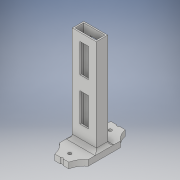
# Autodesk Inventor part: Pizza1
Saved by Autodesk Inventor 2018.2 (Build 222227000, 227)
## iProperties
Created: 2018-03-29
Part Number: Pizza1
Material: Generic
Document SubType Name: Modeling
Designer: MIABo
Density: 1 g/cm^3
Appearance: Default
Author: MIABo
## iProperties of the stored document Pizza1_3DPrint.ipt
Created: 2018-03-29
Part Number: Pizza1_3DPrint
Material: Generic
Document SubType Name: Modeling
Designer: MIABo
Density: 1 g/cm^3
Appearance: Default
Author: MIABo
Autodesk Inventor part; units mm, degrees
ref_plane "YZ Plane" through (0, 0, 0) normal (1, 0, 0) x (0, 1, 0)
ref_plane "XZ Plane" through (0, 0, 0) normal (0, 1, 0) x (-1, 0, 0)
ref_plane "XY Plane" through (0, 0, 0) normal (0, 0, 1) x (1, 0, 0)
sketch "Sketch1" plane through (0, 0, 0) normal (0, 1, 0) x (-1, 0, 0)
  line L0 (12.7, 33.3375) -> (-12.7, 33.3375)
  line L1 (-12.7, 33.3375) -> (-12.7, -33.3375)
  line L2 (-12.7, -33.3375) -> (12.7, -33.3375)
  line L3 (12.7, -33.3375) -> (12.7, 33.3375)
  line L4 (12.7, 33.3375) -> (-12.7, -33.3375) construction
  line L5 (-12.7, 33.3375) -> (12.7, -33.3375) construction
  point P0 (0, 0)
  dimension "d0" = 25.4
  dimension "d1" = 66.675
  constraints: 12 end point, 2 midpoint, 2 parallel, 1 horizontal, 1 perpendicular
  measures "d0" distance of L2.end L1.end
  measures "d1" distance of L1.end L0.end
extrude "Extrusion1" add sketch "Sketch1" along normal blind 5.08
sketch "Sketch3" plane through (0, 5.08, 0) normal (0, 1, 0) x (1, 0, 0)
  line L0 (-10.541, 5.08) -> (10.541, 5.08)
  line L1 (10.541, 5.08) -> (10.541, -5.08)
  line L2 (10.541, -5.08) -> (-10.541, -5.08)
  line L3 (-10.541, -5.08) -> (-10.541, 5.08)
  line L4 (-10.541, 5.08) -> (10.541, -5.08) construction
  line L5 (10.541, 5.08) -> (-10.541, -5.08) construction
  point P0 (0, 0)
  dimension "d8" = 21.082
  dimension "d9" = 10.16
  constraints: 12 end point, 2 midpoint, 2 parallel, 1 horizontal, 1 perpendicular
  measures "d8" distance of L1.end L2.end
  measures "d9" distance of L0.end L1.end
extrude "Extrusion3" add sketch "Sketch3" along normal blind 96.8375
sketch "Sketch2" plane through (0, 5.08, 0) normal (0, 1, 0) x (1, 0, 0)
  line L0 (-9.271, -3.81) -> (9.271, -3.81)
  line L1 (9.271, -3.81) -> (9.271, 3.81)
  line L2 (9.271, 3.81) -> (-9.271, 3.81)
  line L3 (-9.271, 3.81) -> (-9.271, -3.81)
  line L4 (-9.271, -3.81) -> (9.271, 3.81) construction
  line L5 (9.271, -3.81) -> (-9.271, 3.81) construction
  point P0 (0, 0)
  dimension "d4" = 18.542
  dimension "d5" = 7.62
  constraints: 12 end point, 2 midpoint, 2 parallel, 1 horizontal, 1 perpendicular
  measures "d4" distance of L2.end L1.end
  measures "d5" distance of L1.end L0.end
extrude "Extrusion2" cut sketch "Sketch2" along normal through all both and the other way through all
fillet "Fillet1" radius 3.175 4 edges at (0, 5.08, 5.08) (10.541, 5.08, 0) (0, 5.08, -5.08) (-10.541, 5.08, 0)
sketch "Sketch5" plane through (0, 101.9175, 0) normal (0, 1, 0) x (1, 0, 0)
  line L0 (-19.05, 12.7) -> (19.05, 12.7)
  line L1 (19.05, 12.7) -> (19.05, -12.7)
  line L2 (19.05, -12.7) -> (-19.05, -12.7)
  line L3 (-19.05, -12.7) -> (-19.05, 12.7)
  line L4 (-19.05, 12.7) -> (19.05, -12.7) construction
  line L5 (19.05, 12.7) -> (-19.05, -12.7) construction
  point P0 (0, 0)
  constraints: 12 end point, 2 midpoint, 2 parallel, 1 horizontal, 1 perpendicular
extrude "Extrusion5" cut sketch "Sketch5" against normal blind 12.7
sketch "Sketch6" plane through (0, 5.08, 0) normal (0, 1, 0) x (1, 0, 0)
  point P0 (0, 0)
sketch "Sketch7" plane through (0, 5.08, 0) normal (0, 1, 0) x (1, 0, 0)
  line L0 (12.7, 33.3375) -> (-12.7, 33.3375) projected
  line L1 (12.7, -33.3375) -> (12.7, 33.3375) projected
  arc A0 (6.35, 33.3375) -> (12.7, 14.0352) centre (24.8324, 28.7221) ccw
  line L2 (-12.7, 33.3375) -> (-12.7, -33.3375) projected
  arc A1 (-12.7, 14.0352) -> (-6.35, 33.3375) centre (-24.8324, 28.7221) ccw
  line L3 (-12.7, -33.3375) -> (12.7, -33.3375) projected
  arc A2 (-6.35, -33.3375) -> (-12.7, -14.0352) centre (-24.8324, -28.7221) ccw
  arc A3 (12.7, -14.0352) -> (6.35, -33.3375) centre (24.8324, -28.7221) ccw
  line L4 (12.7, -14.0352) -> (12.7, -33.3375)
  line L5 (12.7, -33.3375) -> (6.35, -33.3375)
  line L6 (-6.35, -33.3375) -> (-12.7, -33.3375)
  line L7 (-12.7, -14.0352) -> (-12.7, -33.3375)
  line L8 (-12.7, 14.0352) -> (-12.7, 33.3375)
  line L9 (-6.35, 33.3375) -> (-12.7, 33.3375)
  line L10 (6.35, 33.3375) -> (12.7, 33.3375)
  line L11 (12.7, 14.0352) -> (12.7, 33.3375)
  point P0 (0, 0)
  dimension "d62" = 20.32
  dimension "d63" = 19.05
  dimension "d64" = 20.32
  dimension "d65" = 19.05
  dimension "d68" = 20.32
  dimension "d69" = 19.05
  dimension "d70" = 19.05
  constraints: 16 end point, 8 point on circle, 6 collinear, 6 point on line, 4 centre point, 1 horizontal, 1 perpendicular
  measures "d62" distance of L10.start L11.start
  measures "d63" radius of A0
  measures "d64" distance of L9.start L8.start
  measures "d65" radius of A1
  measures "d68" distance of L6.start L7.start
  measures "d69" radius of A2
  measures "d70" radius of A3
extrude "Extrusion6" cut sketch "Sketch7" against normal blind 25.4 contours L1 A0 L0 | A1 L2 L0 | L1 L3 A3 | A2 L3 L2
sketch "Sketch8" plane through (0, 5.08, 0) normal (0, 1, 0) x (1, 0, 0)
  circle A0 centre (0, 25.4) radius 1.4097
  circle A1 centre (0, -25.4) radius 1.4097
  point P0 (0, 0)
  dimension "d73" = 2.8194
  dimension "d74" = 2.8194
  constraints: 2 centre point
  measures "d73" diameter of A0
  measures "d74" diameter of A1
extrude "Extrusion7" cut sketch "Sketch8" against normal blind 25.4
sketch "Sketch9" plane through (-10.541, 8.255, 5.08) normal (0, 0, 1) x (1, 0, 0)
  line L0 (6.7945, 74.0535) -> (14.2875, 74.0535)
  line L1 (14.2875, 74.0535) -> (14.2875, 48.6535)
  line L2 (14.2875, 48.6535) -> (6.7945, 48.6535)
  line L3 (6.7945, 48.6535) -> (6.7945, 74.0535)
  line L4 (6.7945, 74.0535) -> (14.2875, 48.6535) construction
  line L5 (14.2875, 74.0535) -> (6.7945, 48.6535) construction
  line L6 (6.7945, 11.1125) -> (14.2875, 11.1125)
  line L7 (14.2875, 11.1125) -> (14.2875, 36.5125)
  line L8 (14.2875, 36.5125) -> (6.7945, 36.5125)
  line L9 (6.7945, 36.5125) -> (6.7945, 11.1125)
  line L10 (6.7945, 11.1125) -> (14.2875, 36.5125) construction
  line L11 (14.2875, 11.1125) -> (6.7945, 36.5125) construction
  point P0 (10.541, -8.255)
  point P1 (10.541, 61.3535)
  point P2 (10.541, 23.8125)
  dimension "d77" = 25.4
  dimension "d78" = 25.4
  constraints: 24 end point, 4 midpoint, 4 parallel, 2 horizontal, 2 perpendicular
  measures "d77" distance of L0.end L1.end
  measures "d78" distance of L7.end L6.end
extrude "Extrusion8" cut sketch "Sketch9" against normal blind 25.4
sketch "Sketch10" plane through (0, 5.08, 0) normal (0, 1, 0) x (1, 0, 0)
  line L0 (12.7, 8.255) -> (-12.7, 8.255) projected
  line L1 (0, 8.255) -> (0, 24.765)
  line L2 (0, 24.765) -> (0, 8.255)
  line L3 (-12.7, -8.255) -> (12.7, -8.255) projected
  line L4 (0, -8.255) -> (0, -24.765)
  line L5 (0, -24.765) -> (0, -8.255)
  line L6 (25.4, -49.7649) -> (25.4, -24.765)
  line L7 (25.4, -24.765) -> (-25.4, -24.765)
  line L8 (-25.4, -24.765) -> (-25.4, -49.7649)
  line L9 (-25.4, -49.7649) -> (25.4, -49.7649)
  line L10 (25.4, -49.7649) -> (-25.4, -24.765) construction
  line L11 (25.4, -24.765) -> (-25.4, -49.7649) construction
  line L12 (-17.4625, 50.9042) -> (-17.4625, 24.765)
  line L13 (-17.4625, 24.765) -> (17.4625, 24.765)
  line L14 (17.4625, 24.765) -> (17.4625, 50.9042)
  line L15 (17.4625, 50.9042) -> (-17.4625, 50.9042)
  line L16 (-17.4625, 50.9042) -> (17.4625, 24.765) construction
  line L17 (-17.4625, 24.765) -> (17.4625, 50.9042) construction
  point P0 (0, 0)
  point P1 (0, -37.2649)
  point P2 (0, 37.8346)
  dimension "d81" = 16.51
  dimension "d82" = 16.51
  constraints: 32 end point, 6 midpoint, 5 parallel, 3 perpendicular, 2 vertical, 1 collinear, 1 point on line
  measures "d81" distance of L1.start L1.end
  measures "d82" distance of L4.start L4.end
extrude "Extrusion9" cut sketch "Sketch10" against normal blind 25.4
sketch "Sketch11" plane through (0, 5.08, 0) normal (0, 1, 0) x (1, 0, 0)
  circle A0 centre (0, 17.78) radius 1.4097
  circle A1 centre (0, -17.78) radius 1.4097
  point P0 (0, 0)
  dimension "d85" = 2.8194
  dimension "d86" = 2.8194
  constraints: 2 centre point
  measures "d85" diameter of A0
  measures "d86" diameter of A1
extrude "Extrusion10" cut sketch "Sketch11" against normal blind 25.4
body "Solid1"
